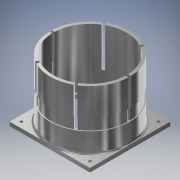
# Autodesk Inventor part: Cup_Dispenser_Flip_Flop
Saved by Autodesk Inventor 2016 (Build 200138000, 138)
## iProperties
Created: 2015-07-03
Part Number: Cup_Dispenser_Flip_Flop
Material: Generic
Document SubType Name: Modeling
Designer: bastli
Density: 1 g/cm^3
Appearance: Steel - Polished
Author: bastli
Autodesk Inventor part; units mm, degrees
ref_plane "YZ Plane" through (0, 0, 0) normal (1, 0, 0) x (0, 1, 0)
ref_plane "XZ Plane" through (0, 0, 0) normal (0, 1, 0) x (-1, 0, 0)
ref_plane "XY Plane" through (0, 0, 0) normal (0, 0, 1) x (1, 0, 0)
sketch "Sketch1" plane through (0, 0, 0) normal (0, 0, 1) x (1, 0, 0)
  circle A0 centre (0, 0) radius 37.5 projected
  circle A1 centre (0, 0) radius 40.5
  point P0 (0, 0)
  dimension "d0" = 3
  constraints: 1 centre point
  measures "d0" radial gap between concentric circles of A0 A1
extrude "Extrusion1" add sketch "Sketch1" against normal blind 60
sketch "Sketch8" plane through (0, 0, 0) normal (0, 0, 1) x (1, 0, 0)
  line L0 (0, 0) -> (-46.6973, 0) construction
  line L1 (0, 0) -> (-40.4753, 1.4134) construction
  circle A0 centre (0, 0) radius 40.5 projected
  line L2 (0, 0) -> (-40.4753, -1.4134) construction
  circle A1 centre (0, 0) radius 37.5 projected
  line L3 (-37.4772, -1.3087) -> (-40.4753, -1.4134)
  line L4 (-37.4772, 1.3087) -> (-40.4753, 1.4134)
  dimension "d30" = 4
  constraints: 10 end point, 4 point on circle, 2 collinear, 2 point on line, 1 horizontal, 1 other
  measures "d30" angle of L1 L2
extrude "Extrusion9" cut sketch "Sketch8" against normal blind 40 contours L4 A1 L3 A0 picked at (-39.4973, -0.1454)
pattern_circular "Circular Pattern2" count 6 over 360 about axis through (0, 0, 0) along (0, 0, -1) of "Extrusion9"
sketch "Sketch9" plane through (21.4617, -34.3459, -40) normal (0, 0, 1) x (0.848, 0.5299, 0)
  circle A0 centre (0, 40.5) radius 37.5 construction
  circle A1 centre (0, 40.5) radius 40.5 projected
  circle A2 centre (0, 40.5) radius 39.5
  point P0 (0, 40.5)
  dimension "d36" = 1
  constraints: 1 centre point
  measures "d36" radial gap between concentric circles of A1 A2
extrude "Extrusion10" cut sketch "Sketch9" along normal blind 12
sketch "Sketch10" plane through (0, 0, -60) normal (0, 0, -1) x (-1, 0, 0)
  line L0 (41, -41) -> (-41, -41)
  line L1 (-41, -41) -> (-41, 41)
  line L2 (-41, 41) -> (41, 41)
  line L3 (41, 41) -> (41, -41)
  line L4 (41, -41) -> (-41, 41) construction
  line L5 (-41, -41) -> (41, 41) construction
  circle A0 centre (0, 0) radius 37.5 construction
  circle A1 centre (0, 0) radius 35.5
  point P0 (0, 0)
  dimension "d39" = 82
  dimension "d40" = 82
  dimension "d41" = 2
  constraints: 12 end point, 2 midpoint, 2 parallel, 1 centre point, 1 horizontal, 1 perpendicular
  measures "d39" distance of L1.end L2.end
  measures "d40" distance of L0.end L1.end
  measures "d41" radial gap between concentric circles of A0 A1
extrude "Extrusion11" add sketch "Sketch10" along normal blind 4
sketch "Sketch11" plane through (0, 0, -60) normal (0, 0, 1) x (1, 0, 0)
  line L0 (-41, 41) -> (-41, -41) construction
  line L1 (-41, -41) -> (41, -41) construction
  line L2 (41, -41) -> (41, 41) construction
  line L3 (41, 41) -> (-41, 41) construction
  line L4 (-35, -35) -> (-35, 35) construction
  line L5 (-35, 35) -> (35, 35) construction
  line L6 (35, 35) -> (35, -35) construction
  line L7 (35, -35) -> (-35, -35) construction
  point P0 (0, 0)
  dimension "d44" = 6
  constraints: 8 end point, 4 coincident, 3 other
  measures "d44" distance between parallel lines of L0 L4
hole "Hole1" at (-35, -35, -60) at (-35, 35, -60) at (35, 35, -60) at (35, -35, -60) direction (0, 0, -1) diameter 3 end through all
fillet "Fillet2" radius 2 1 edges at (-40.5, 0, -60)
sketch "Sketch7" plane through (0, 0, -5) normal (0, 0, -1) x (-1, 0, 0)
  circle A0 centre (0, 0) radius 40.5 projected
  circle A1 centre (0, 0) radius 39.5
  point P0 (0, 0)
  dimension "d27" = 1
  constraints: 1 centre point
  measures "d27" radial gap between concentric circles of A0 A1
body "Solid1"
